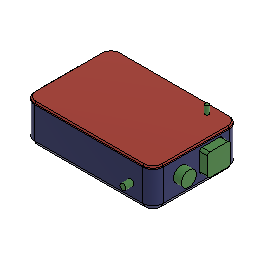
M4xxxATMega (Autodesk Fusion 360 design; units mm, degrees)
Autodesk Fusion 360 part; units mm, degrees
sketch "Sketch2" plane through (0, 0, 0) normal (0, 0, 1) x (1, 0, 0) in component "PCB"
  line L0 (50, -32.5) -> (-50, -32.5)
  line L1 (-50, -32.5) -> (-50, 32.5)
  line L2 (-50, 32.5) -> (50, 32.5)
  line L3 (50, 32.5) -> (50, -32.5)
  line L4 (50, -32.5) -> (-50, 32.5) construction
  line L5 (-50, -32.5) -> (50, 32.5) construction
  line L6 (0, 0) -> (0, 32.5) construction
  line L7 (0, 0) -> (-50, 0) construction
  circle A0 centre (-45, 27.5) radius 1.6
  circle A1 centre (45, 27.5) radius 1.6
  circle A2 centre (45, -27.5) radius 1.6
  circle A3 centre (-45, -27.5) radius 1.6
  line L8 (50, -21.75) -> (26, -21.75)
  line L9 (26, -21.75) -> (26, -3.25)
  line L10 (26, -3.25) -> (50, -3.25)
  line L11 (50, -3.25) -> (50, -21.75)
  line L12 (50, -21.75) -> (26, -3.25) construction
  line L13 (26, -21.75) -> (50, -3.25) construction
  line L14 (50, 1.75) -> (30, 1.75)
  line L15 (30, 1.75) -> (30, 23.25)
  line L16 (30, 23.25) -> (50, 23.25)
  line L17 (50, 23.25) -> (50, 1.75)
  line L18 (50, 1.75) -> (30, 23.25) construction
  line L19 (30, 1.75) -> (50, 23.25) construction
  line L20 (-42, -15) -> (-50, -15)
  line L21 (-50, -15) -> (-50, 15)
  line L22 (-50, 15) -> (-42, 15)
  line L23 (-42, 15) -> (-42, -15)
  line L24 (-42, -15) -> (-50, 15) construction
  line L25 (-50, -15) -> (-42, 15) construction
  circle A4 centre (35, 27.5) radius 1.6
  line L26 (38.5, -32.5) -> (31.5, -32.5)
  line L27 (31.5, -32.5) -> (31.5, -25.5)
  line L28 (31.5, -25.5) -> (38.5, -25.5)
  line L29 (38.5, -25.5) -> (38.5, -32.5)
  line L30 (38.5, -32.5) -> (31.5, -25.5) construction
  line L31 (31.5, -32.5) -> (38.5, -25.5) construction
  line L32 (50, 23.25) -> (51.01, 23.25)
  line L33 (51.01, 23.25) -> (51.01, 1.75)
  line L34 (51.01, 1.75) -> (50, 1.75)
  line L35 (50, 1.75) -> (50, 23.25)
  point P0 (38, -12.5)
  point P1 (40, 12.5)
  point P2 (-46, 0)
  point P3 (35, -29)
  dimension "d1" = 100
  dimension "d2" = 65
  dimension "d3" = 5
  dimension "d4" = 5
  dimension "d5" = 3.2
  dimension "d6" = 24
  dimension "d7" = 18.5
  dimension "d8" = 45
  dimension "d9" = 21.5
  dimension "d10" = 20
  dimension "d11" = 20
  dimension "d12" = 30
  dimension "d13" = 8
  dimension "d14" = 3.2
  dimension "d15" = 85
  dimension "d16" = 7
  dimension "d17" = 7
  dimension "d74" = 1.01
  constraint perpendicular L0 L1
  constraint parallel L0 L2
  constraint parallel L1 L3
  constraint horizontal L0
  constraint coincident L4 L6.start
  constraint coincident L5 L6.start
  constraint coincident L6.start L7.start
  constraint midpoint L2 L6.end
  constraint midpoint L1 L7.end
  constraint symmetric L6 A0 A1
  constraint symmetric L7 A0 A3
  constraint symmetric L7 A1 A2
  constraint perpendicular L8 L9
  constraint parallel L8 L10
  constraint parallel L9 L11
  constraint horizontal L8
  constraint coincident L12 P0
  constraint coincident L13 P0
  constraint coincident L3 L10.end
  constraint perpendicular L14 L15
  constraint parallel L14 L16
  constraint parallel L15 L17
  constraint horizontal L14
  constraint coincident L18 P1
  constraint coincident L19 P1
  constraint coincident L3 L14.start
  constraint perpendicular L20 L21
  constraint parallel L20 L22
  constraint parallel L21 L23
  constraint horizontal L20
  constraint coincident L24 P2
  constraint coincident L25 P2
  constraint coincident L1 L20.end
  constraint horizontal A0.centre A4.centre
  constraint perpendicular L26 L27
  constraint parallel L26 L28
  constraint parallel L27 L29
  constraint horizontal L26
  constraint coincident L30 P3
  constraint coincident L31 P3
  constraint coincident L0 L26.start
  constraint vertical A4.centre P3
  constraint coincident L7 P2
  constraint horizontal L32
  constraint vertical L33
  constraint horizontal L34
  constraint vertical L35
  constraint collinear L14 L34
  measures "d1" distance of L1.end L2.end
  measures "d2" distance of L0.end L1.end
  measures "d3" distance of L2 A0.centre
  measures "d4" distance of L1 A0.centre
  measures "d5" diameter of A0
  measures "d6" distance of L9.end L10.end
  measures "d7" distance of L8.end L9.end
  measures "d8" distance of L2 P0
  measures "d9" distance of L14.end L15.end
  measures "d10" distance of L15.end L16.end
  measures "d11" distance of L2 P1
  measures "d12" distance of L20.end L21.end
  measures "d13" distance of L21.end L22.end
  measures "d14" diameter of A4
  measures "d15" distance of L1 A4.centre
  measures "d16" distance of L26.end L27.end
  measures "d17" distance of L27.end L28.end
  measures "d74" distance of L16.end L32.end
extrude "Extrude1" add sketch "Sketch2" against normal blind 1.6 contours L0 L1 L2 L3 L8 L9 L10 L14 L15 L16 L20 L22 L23 L27 L28 L29 | L0 L26 L27 L28 L29 | L3 L8 L9 L10 L11 | L3 L14 L15 L16 L17 L35 | L1 L20 L21 L22 L23 | A4 makes body 1 in component "PCB"
extrude "Extrude2" add sketch "Sketch2" along normal blind 16 contours L1 L20 L21 L22 L23 bodies 1 in component "PCB"
extrude "Extrude3" add sketch "Sketch2" along normal blind 8 contours L0 L26 L27 L28 L29 bodies 1 in component "PCB"
extrude "Extrude4" add sketch "Sketch2" along normal blind 15.5 contours L3 L8 L9 L10 L11 bodies 1 in component "PCB"
extrude "Extrude5" add sketch "Sketch2" along normal blind 21 contours L3 L14 L15 L16 L17 L35 | L3 L17 L32 L33 L34 L35 bodies 1 in component "PCB"
extrude "Extrude6" add sketch "Sketch2" along normal blind 30 contours A4 bodies 1 in component "PCB"
sketch "Sketch3" plane through (-50, 0, 0) normal (-1, 0, 0) x (0, -1, 0) in component "PCB"
  line L0 (32.5, 0) -> (15, 0)
  line L1 (15, 0) -> (15, 16)
  line L2 (15, 16) -> (-15, 16)
  line L3 (-15, 16) -> (-15, 0)
  line L4 (-15, 0) -> (-32.5, 0)
  line L5 (-32.5, 0) -> (-32.5, -1.6)
  line L6 (-32.5, -1.6) -> (32.5, -1.6)
  line L7 (32.5, -1.6) -> (32.5, 0)
  line L8 (-15, 12) -> (15, 12)
  dimension "d30" = 4
  constraint coincident L3 L8.start
  constraint coincident L1 L8.end
  constraint perpendicular L1 L8
  measures "d30" distance of L2 L8
extrude "Extrude7" add sketch "Sketch3" along normal blind 10 contours L1 L2 L3 L8 bodies 1 in component "PCB"
sketch "Sketch4" plane through (0, -32.5, 0) normal (0, -1, 0) x (1, 0, 0) in component "PCB"
  line L0 (50, 0) -> (38.5, 0)
  line L1 (38.5, 0) -> (38.5, 8)
  line L2 (38.5, 8) -> (31.5, 8)
  line L3 (31.5, 8) -> (31.5, 0)
  line L4 (31.5, 0) -> (-50, 0)
  line L5 (-50, 0) -> (-50, -1.6)
  line L6 (-50, -1.6) -> (50, -1.6)
  line L7 (50, -1.6) -> (50, 0)
  circle A0 centre (35, 5.5) radius 2.5
  point P0 (35, 0)
  dimension "d33" = 5
  dimension "d73" = 5.5
  constraint vertical A0.centre P0
  measures "d33" diameter of A0
  measures "d73" distance of A0.centre P0
extrude "Extrude8" add sketch "Sketch4" along normal blind 10 contours A0 bodies 1 in component "PCB"
sketch "Sketch5" plane through (50, 0, 0) normal (1, 0, 0) x (0, 1, 0) in component "PCB"
  line L0 (32.5, 0) -> (23.25, 0)
  line L1 (-3.25, 0) -> (-3.25, 15.5)
  line L2 (-3.25, 15.5) -> (-21.75, 15.5)
  line L3 (-21.75, 15.5) -> (-21.75, 0)
  line L4 (-21.75, 0) -> (-32.5, 0)
  line L5 (-32.5, 0) -> (-32.5, -1.6)
  line L6 (-32.5, -1.6) -> (32.5, -1.6)
  line L7 (32.5, -1.6) -> (32.5, 0)
  circle A0 centre (-12.5, 9) radius 6.25
  line L8 (22, 1) -> (3, 1)
  line L9 (3, 1) -> (3, 19.5)
  line L10 (3, 19.5) -> (22, 19.5)
  line L11 (22, 19.5) -> (22, 1)
  line L12 (22, 1) -> (3, 19.5) construction
  line L13 (3, 1) -> (22, 19.5) construction
  line L14 (23.25, 0) -> (1.75, 0)
  line L15 (1.75, 0) -> (-3.25, 0)
  line L16 (12.5, 0) -> (12.5, 10.25) construction
  point P0 (-12.5, 0)
  point P1 (12.5, 10.25)
  point P2 (12.5, 0)
  dimension "d36" = 12.5
  dimension "d37" = 9
  dimension "d41" = 1
  dimension "d77" = 19
  constraint vertical A0.centre P0
  constraint perpendicular L8 L9
  constraint parallel L8 L10
  constraint parallel L9 L11
  constraint horizontal L8
  constraint coincident L12 P1
  constraint coincident L13 P1
  constraint vertical P1 P2
  constraint coincident P2 L16.start
  constraint midpoint L13 P1
  measures "d36" diameter of A0
  measures "d37" distance of A0.centre P0
  measures "d41" distance of L8 P2
  measures "d77" distance of L9.end L10.end
extrude "Extrude9" add sketch "Sketch5" along normal blind 10 contours A0 | L8 L9 L10 L11 bodies 1 in component "PCB"
fillet "Fillet1" radius 2 4 edges at (55.505, 22, 19.5) (55.505, 3, 19.5) (55.505, 22, 1) (55.505, 3, 1) on bodies 1 in component "PCB"
fillet "Fillet1" radius 5 4 edges at (50, 32.5, -0.8) (50, -32.5, -0.8) (-50, 32.5, -0.8) (-50, -32.5, -0.8) on bodies 1 in component "PCB"
ref_plane "WorkPlane1" through (0, 0, -6.6) normal (0, 0, -1) x (-1, 0, 0) in component "Base"
sketch "Sketch1" plane through (0, 0, -6.6) normal (0, 0, -1) x (1, 0, 0) in component "Base"
  arc A0 (-45, 32.5) -> (-50, 27.5) centre (-45, 27.5) ccw construction
  line L0 (-50, 27.5) -> (-50, -27.5) construction
  arc A1 (-50, -27.5) -> (-45, -32.5) centre (-45, -27.5) ccw construction
  line L1 (-45, -32.5) -> (45, -32.5) construction
  arc A2 (45, -32.5) -> (50, -27.5) centre (45, -27.5) ccw construction
  line L2 (50, -27.5) -> (50, 27.5) construction
  arc A3 (50, 27.5) -> (45, 32.5) centre (45, 27.5) ccw construction
  line L3 (45, 32.5) -> (-45, 32.5) construction
  circle A4 centre (45, 27.5) radius 1.6 construction
  circle A5 centre (-45, -27.5) radius 1.6 construction
  circle A6 centre (-45, 27.5) radius 1.6 construction
  circle A7 centre (45, -27.5) radius 1.6 construction
  line L4 (-51, 27.5) -> (-51, -27.5)
  arc A8 (-51, -27.5) -> (-45, -33.5) centre (-45, -27.5) ccw
  line L5 (-45, -33.5) -> (45, -33.5)
  arc A9 (45, -33.5) -> (51, -27.5) centre (45, -27.5) ccw
  line L6 (51, -27.5) -> (51, 27.5)
  arc A10 (51, 27.5) -> (45, 33.5) centre (45, 27.5) ccw
  line L7 (45, 33.5) -> (-45, 33.5)
  arc A11 (-45, 33.5) -> (-51, 27.5) centre (-45, 27.5) ccw
  line L8 (-53.4, 27.5) -> (-53.4, -27.5)
  arc A12 (-53.4, -27.5) -> (-45, -35.9) centre (-45, -27.5) ccw
  line L9 (-45, -35.9) -> (45, -35.9)
  arc A13 (45, -35.9) -> (53.4, -27.5) centre (45, -27.5) ccw
  line L10 (53.4, -27.5) -> (53.4, 27.5)
  arc A14 (53.4, 27.5) -> (45, 35.9) centre (45, 27.5) ccw
  line L11 (45, 35.9) -> (-45, 35.9)
  arc A15 (-45, 35.9) -> (-53.4, 27.5) centre (-45, 27.5) ccw
  circle A16 centre (-45, -27.5) radius 4
  line L12 (-43.5, -27.5) -> (-44.25, -26.201)
  line L13 (-44.25, -26.201) -> (-45.75, -26.201)
  line L14 (-45.75, -26.201) -> (-46.5, -27.5)
  line L15 (-46.5, -27.5) -> (-45.75, -28.799)
  line L16 (-45.75, -28.799) -> (-44.25, -28.799)
  line L17 (-44.25, -28.799) -> (-43.5, -27.5)
  line L18 (0, 0) -> (0, -33.5) construction
  line L19 (0, 0) -> (-51, 0) construction
  circle A17 centre (-45, 27.5) radius 4
  line L20 (-45.75, 28.799) -> (-44.25, 28.799)
  line L21 (-46.5, 27.5) -> (-45.75, 28.799)
  line L22 (-45.75, 26.201) -> (-46.5, 27.5)
  line L23 (-44.25, 26.201) -> (-45.75, 26.201)
  line L24 (-43.5, 27.5) -> (-44.25, 26.201)
  line L25 (-44.25, 28.799) -> (-43.5, 27.5)
  circle A18 centre (45, 27.5) radius 4
  line L26 (44.25, 26.201) -> (45.75, 26.201)
  line L27 (43.5, 27.5) -> (44.25, 26.201)
  line L28 (44.25, 28.799) -> (43.5, 27.5)
  line L29 (45.75, 28.799) -> (44.25, 28.799)
  line L30 (46.5, 27.5) -> (45.75, 28.799)
  line L31 (45.75, 26.201) -> (46.5, 27.5)
  line L32 (44.25, -26.201) -> (45.75, -26.201)
  line L33 (43.5, -27.5) -> (44.25, -26.201)
  line L34 (44.25, -28.799) -> (43.5, -27.5)
  line L35 (45.75, -28.799) -> (44.25, -28.799)
  line L36 (46.5, -27.5) -> (45.75, -28.799)
  line L37 (45.75, -26.201) -> (46.5, -27.5)
  circle A19 centre (45, -27.5) radius 4
  point P0 (-45, -27.5)
  dimension "d46" = 1
  dimension "d47" = 3.4
  dimension "d55" = 8
  dimension "d56" = 1.5
  constraint concentric A1 A16
  constraint coincident P0 A1.centre
  constraint coincident L18.start L19.start
  constraint midpoint L5 L18.end
  constraint midpoint L4 L19.end
  constraint horizontal L13
  constraint symmetric A16 L19 A17
  constraint symmetric L12.start L19 L24.start
  constraint symmetric L12.end L19 L23.start
  constraint symmetric L13.end L19 L22.start
  constraint symmetric L14.end L19 L21.start
  constraint symmetric L15.end L19 L20.start
  constraint symmetric L16.end L19 L20.end
  constraint symmetric A16 L18 A19
  constraint symmetric L12.start L18 L33.start
  constraint symmetric L12.end L18 L32.start
  constraint symmetric L13.end L18 L32.end
  constraint symmetric L14.end L18 L36.start
  constraint symmetric L15.end L18 L35.start
  constraint symmetric L16.end L18 L34.start
  constraint symmetric L18 A17 A18
  constraint symmetric L18 L20.start L29.start
  constraint symmetric L18 L20.end L28.start
  constraint symmetric L18 L21.start L30.start
  constraint symmetric L18 L22.start L26.end
  constraint symmetric L18 L23.start L26.start
  constraint symmetric L18 L24.start L27.start
  measures "d55" diameter of A16
  measures "d56" distance of L12.start P0
extrude "Extrude1'" add sketch "Sketch1" along normal blind 1.6 separate body contours L4 A8 L5 A9 L6 A10 L7 A11 | L8 A12 L9 A13 L10 A14 L11 A15 | A16 | L12 L13 L14 L15 L16 L17 | A17 | L20 L21 L22 L23 L24 L25 | A18 | L26 L27 L28 L29 L30 L31 | L32 L33 L34 L35 L36 L37 | A19 makes body 2 in component "Base"
extrude "Extrude2'" add sketch "Sketch1" against normal blind 28 contours L8 A12 L9 A13 L10 A14 L11 A15 bodies 2 in component "Base"
extrude "Extrude3'" add sketch "Sketch1" against normal blind 5 contours A16 | A17 | A18 | A19 bodies 2 in component "Base"
chamfer "Chamfer1" distance 1 angle 45 16 edges at (51, 0, -6.6) (49.2426, 31.7426, -6.6) (0, 33.5, -6.6) (-49.2426, 31.7426, -6.6) (-51, 0, -6.6) (-49.2426, -31.7426, -6.6) (0, -33.5, -6.6) (49.2426, -31.7426, -6.6) (41.2707, -26.0535, -6.6) (-48.7293, -26.0535, -6.6) (41.2707, 28.9465, -6.6) (-48.7293, 28.9465, -6.6) (-48.7293, 26.0535, -1.6) (41.2707, 26.0535, -1.6) (-48.7293, -28.9465, -1.6) (41.2707, -28.9465, -1.6) on bodies 2 in component "Base"
chamfer "Chamfer2" distance 2 angle 60 8 edges at (-53.4, 0, -8.2) (-50.9397, 33.4397, -8.2) (0, 35.9, -8.2) (50.9397, 33.4397, -8.2) (53.4, 0, -8.2) (50.9397, -33.4397, -8.2) (0, -35.9, -8.2) (-50.9397, -33.4397, -8.2) measured on face at (-15, 11.9667, -8.2) measured on face at (-15, 11.9667, -8.2) measured on face at (-15, 11.9667, -8.2) measured on face at (-15, 11.9667, -8.2) measured on face at (-15, 11.9667, -8.2) measured on face at (-15, 11.9667, -8.2) measured on face at (-15, 11.9667, -8.2) measured on face at (-15, 11.9667, -8.2) on bodies 2 in component "Base"
sketch "Sketch2 (2)" plane through (0, 0, 21.4) normal (0, 0, 1) x (-1, 0, 0) in component "Lid"
  arc A0 (51, 27.5) -> (45, 33.5) centre (45, 27.5) ccw
  line L0 (51, 27.5) -> (51, -27.5)
  arc A1 (45, -33.5) -> (51, -27.5) centre (45, -27.5) ccw
  line L1 (45, -33.5) -> (-45, -33.5)
  arc A2 (-51, -27.5) -> (-45, -33.5) centre (-45, -27.5) ccw
  line L2 (-51, -27.5) -> (-51, 27.5)
  arc A3 (-45, 33.5) -> (-51, 27.5) centre (-45, 27.5) ccw
  line L3 (-45, 33.5) -> (45, 33.5)
  arc A4 (53.4, 27.5) -> (45, 35.9) centre (45, 27.5) ccw
  line L4 (45, 35.9) -> (-45, 35.9)
  arc A5 (-45, 35.9) -> (-53.4, 27.5) centre (-45, 27.5) ccw
  line L5 (-53.4, 27.5) -> (-53.4, -27.5)
  arc A6 (-53.4, -27.5) -> (-45, -35.9) centre (-45, -27.5) ccw
  line L6 (-45, -35.9) -> (45, -35.9)
  arc A7 (45, -35.9) -> (53.4, -27.5) centre (45, -27.5) ccw
  line L7 (53.4, -27.5) -> (53.4, 27.5)
  arc A8 (-48.6, -27.5) -> (-45, -31.1) centre (-45, -27.5) ccw
  line L8 (45, -31.1) -> (-45, -31.1)
  arc A9 (45, -31.1) -> (48.6, -27.5) centre (45, -27.5) ccw
  line L9 (48.6, 27.5) -> (48.6, -27.5)
  arc A10 (48.6, 27.5) -> (45, 31.1) centre (45, 27.5) ccw
  line L10 (-45, 31.1) -> (45, 31.1)
  arc A11 (-45, 31.1) -> (-48.6, 27.5) centre (-45, 27.5) ccw
  line L11 (-48.6, -27.5) -> (-48.6, 27.5)
  dimension "d64" = 2.4
extrude "Extrude1''" add sketch "Sketch2 (2)" against normal blind 6 separate body contours A0 L0 A1 L1 A2 L2 A3 L3 makes body 3 in component "Lid"
extrude "Extrude2''" add sketch "Sketch2 (2)" along normal blind 2 contours A0 L0 A1 L1 A2 L2 A3 L3 | A4 L4 A5 L5 A6 L6 A7 L7 | A8 L8 A9 L9 A10 L10 A11 L11 bodies 3 in component "Lid"
chamfer "Chamfer1'" distance 1 angle 45 8 edges at (53.4, 0, 23.4) (50.9397, 33.4397, 23.4) (0, 35.9, 23.4) (-50.9397, 33.4397, 23.4) (-53.4, 0, 23.4) (-50.9397, -33.4397, 23.4) (0, -35.9, 23.4) (50.9397, -33.4397, 23.4) measured on face at (-15, 11.9667, 23.4) measured on face at (-15, 11.9667, 23.4) measured on face at (-15, 11.9667, 23.4) measured on face at (-15, 11.9667, 23.4) measured on face at (-15, 11.9667, 23.4) measured on face at (-15, 11.9667, 23.4) measured on face at (-15, 11.9667, 23.4) measured on face at (-15, 11.9667, 23.4) on bodies 3 in component "Lid"
chamfer "Chamfer2'" distance 0.4 angle 60 8 edges at (-51, 0, 15.4) (-49.2426, 31.7426, 15.4) (0, 33.5, 15.4) (49.2426, 31.7426, 15.4) (51, 0, 15.4) (49.2426, -31.7426, 15.4) (0, -33.5, 15.4) (-49.2426, -31.7426, 15.4) measured on face at (-15, -31.9, 15.4) measured on face at (-15, -31.9, 15.4) measured on face at (-15, -31.9, 15.4) measured on face at (-15, -31.9, 15.4) measured on face at (-15, -31.9, 15.4) measured on face at (-15, -31.9, 15.4) measured on face at (-15, -31.9, 15.4) measured on face at (-15, -31.9, 15.4) on bodies 3 in component "Lid"
combine "Combine1" operation cut target body 3 tool bodies 1 keep tools in component "Lid"
chamfer "Chamfer3" distance 2 angle 45 2 edges at (49.6, 1.75, 15.4) (49.6, 23.25, 15.4) on bodies 3 in component "Lid"
chamfer "Chamfer4" distance 0.8 angle 45 1 edges at (33.5083, 26.9214, 21.4) on bodies 3 in component "Lid"
combine "Combine1'" operation cut target body 2 tool bodies 1 keep tools in component "Base"
component "PCB" placed x (1, 0, 0) y (0, 1, 0) z (0, 0, 1) at (0, 0, 0)
component "Base" placed x (1, 0, 0) y (0, 1, 0) z (0, 0, 1) at (0, 0, 0)
component "Lid" placed x (1, 0, 0) y (0, 1, 0) z (0, 0, 1) at (0, 0, 0)
named bodies: "PCB", "Base", "Lid"
